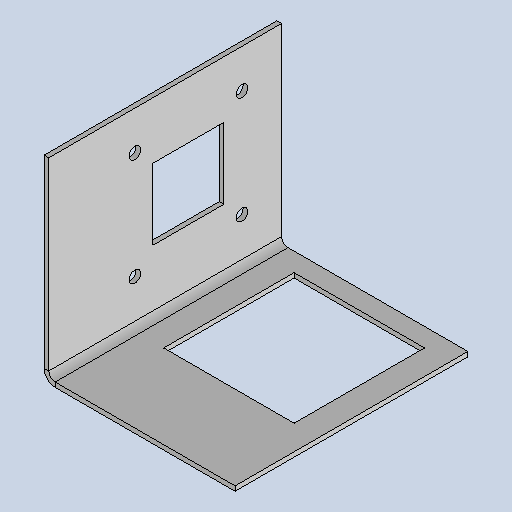
# Autodesk Inventor part: PRS 1200-510 FDS Central tube wall
Saved by Autodesk Inventor 2025.3 (Build 293356030, 356C)
## iProperties
Created: 2025-06-24
Part Number: PRS 1200-510 FDS Central tube wall
Material: Stainless Steel
Document SubType Name: Sheet Metal
Designer: admin
Mass: 193.508 g
Surface Area: 260.557 cm^2
Volume: 24.1885 cm^3
Density: 8 g/cm^3
Flat Pattern Width: 16.2202 cm
Flat Pattern Length: 10 cm
Flat Pattern Area: 162.202 cm^2
Sheet Metal Rule: AISI304 2mm Die16
Sheet Metal Width: 162,202 mm
Sheet Metal Length: 100,000 mm
Sheet Metal Area: 16220,199 mm^2
Appearance: Default
Author: user
Autodesk Inventor part; units mm, degrees
ref_plane "YZ Plane" through (0, 0, 0) normal (1, 0, 0) x (0, 1, 0)
ref_plane "XZ Plane" through (0, 0, 0) normal (0, 1, 0) x (-1, 0, 0)
ref_plane "XY Plane" through (0, 0, 0) normal (0, 0, 1) x (1, 0, 0)
sketch "Sketch1" plane through (0, 0, 0) normal (0, 0, 1) x (1, 0, 0)
  line L0 (-41, -50) -> (41, -50)
  line L1 (41, -50) -> (41, 50)
  line L2 (41, 50) -> (-41, 50)
  line L3 (-41, 50) -> (-41, -50)
  line L4 (-41, -50) -> (41, 50) construction
  line L5 (41, -50) -> (-41, 50) construction
  point P0 (0, 0)
  dimension "d154" = 82
  dimension "d155" = 100
  measures "d154" distance of L1.end L2.end
  measures "d155" distance of L0.end L1.end
extrude "Plate5" add sketch "Sketch1" along normal blind 2
sketch "Sketch7" plane through (-39, -50, 0) normal (-1, 0, 0) x (0, -1, 0)
  line L0 (-100, 0) -> (0, 0)
  line L1 (0, 0) -> (0, 84)
  line L2 (0, 84) -> (-100, 84)
  line L3 (-100, 84) -> (-100, 0)
  constraints: 6 end point, 1 horizontal, 1 perpendicular, 1 vertical
edge flange "Flange3" height 84 angle 90 thickness 2 bend radius 2.75 thickness toward (-1, 0, 0) relief round relief width 2 relief depth 1 edges at (-41, 0, 2) wall of the first edge with corners at (-39, 50, 0) (-39, -50, 0) (-39, -50, 84) (-39, 50, 84)
bend "Bend3"
corner "Corner3"
sketch "Sketch8" plane through (0, 0, 2) normal (0, 0, 1) x (1, 0, 0)
  line L0 (41, 50) -> (41, -50) projected
  line L1 (-36.25, 50) -> (41, 50) projected
  line L2 (30.375, 42) -> (-25.625, 42)
  line L3 (-25.625, 42) -> (-25.625, -14)
  line L4 (-25.625, -14) -> (30.375, -14)
  line L5 (30.375, -14) -> (30.375, 42)
  line L6 (30.375, 42) -> (-25.625, -14) construction
  line L7 (-25.625, 42) -> (30.375, -14) construction
  point P0 (0, 0)
  point P1 (2.375, 14)
  point P2 (2.375, 50)
  dimension "d167" = 56
  dimension "d168" = 56
  dimension "d169" = 8
  constraints: 12 end point, 3 midpoint, 2 parallel, 1 horizontal, 1 perpendicular, 1 vertical alignment
  measures "d167" distance of L4.end L3.end
  measures "d168" distance of L3.end L2.end
  measures "d169" distance between parallel lines of L1 L2
extrude "Cut1" cut sketch "Sketch8" against normal blind 2
sketch "Sketch9" plane through (-41, -50, 84) normal (-1, 0, 0) x (0, 0, 1)
  line L0 (-24.375, 44.75) -> (-54.875, 44.75)
  line L1 (-54.875, 44.75) -> (-54.875, 75.25)
  line L2 (-54.875, 75.25) -> (-24.375, 75.25)
  line L3 (-24.375, 75.25) -> (-24.375, 44.75)
  line L4 (-24.375, 44.75) -> (-54.875, 75.25) construction
  line L5 (-54.875, 44.75) -> (-24.375, 75.25) construction
  circle A0 centre (-16.625, 37) radius 2.5
  circle A1 centre (-62.625, 37) radius 2.5
  circle A2 centre (-62.625, 83) radius 2.5
  circle A3 centre (-16.625, 83) radius 2.5
  circle A4 centre (-39.625, 60) radius 32.5269 construction
  line L6 (-54.875, 44.75) -> (-62.625, 37) construction
  line L7 (-14.125, 34.5) -> (-65.125, 34.5) construction
  line L8 (-65.125, 34.5) -> (-65.125, 85.5) construction
  line L9 (-65.125, 85.5) -> (-14.125, 85.5) construction
  line L10 (-14.125, 85.5) -> (-14.125, 34.5) construction
  line L11 (-14.125, 34.5) -> (-65.125, 85.5) construction
  line L12 (-65.125, 34.5) -> (-14.125, 85.5) construction
  line L13 (-79.25, 100) -> (0, 100) projected
  line L14 (-39.625, 100) -> (-39.625, 60) construction
  circle A5 centre (-62.625, 83) radius 10.9602 construction
  line L15 (-16.625, 37) -> (-62.625, 37) construction
  line L16 (-62.625, 37) -> (-62.625, 83) construction
  line L17 (-62.625, 83) -> (-16.625, 83) construction
  line L18 (-16.625, 83) -> (-16.625, 37) construction
  line L19 (-16.625, 37) -> (-62.625, 83) construction
  line L20 (-62.625, 37) -> (-16.625, 83) construction
  point P0 (-84, 50)
  point P1 (-104.8197, 150.8767)
  point P2 (-104.8197, 150.8767)
  dimension "d181" = 21.9203
  dimension "d174" = 30.5
  dimension "d175" = 30.5
  dimension "d176" = 5
  dimension "d179" = 40
  dimension "d180" = 51
  dimension "d184" = 46
  constraints: 40 end point, 7 midpoint, 6 parallel, 5 centre point, 5 point on line, 4 point on circle, 3 equal radius, 3 horizontal, 3 perpendicular, 2 coincident, 1 tangent, 1 vertical, 3 other
  measures "d174" distance of L3.end L1.start
  measures "d175" distance of L1.start L1.end
  measures "d176" diameter of A0
  measures "d179" distance from line of L14.end L13
  measures "d180" distance of L7.end L8.end
  measures "d184" distance of L17.end L15.start
extrude "Cut2" cut sketch "Sketch9" against normal blind 2
body "Solid3"
